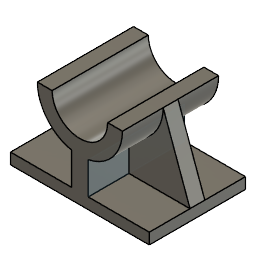
day3 (Autodesk Fusion 360 design; units mm, degrees)
part number: 2026-08-21-14-28-38-884
Autodesk Fusion 360 part; units mm, degrees
sketch "Sketch1" plane through (0, 0, 0) normal (0, 1, 0) x (1, 0, 0)
  line L0 (37.5, 26) -> (-37.5, 26)
  line L1 (-37.5, 26) -> (-37.5, -26)
  line L2 (-37.5, -26) -> (37.5, -26)
  line L3 (37.5, -26) -> (37.5, 26)
  line L4 (37.5, 26) -> (-37.5, -26) construction
  line L5 (-37.5, 26) -> (37.5, -26) construction
  dimension "d1" = 75
  dimension "d2" = 52
  constraint horizontal L0
  constraint perpendicular L0 L1
  constraint parallel L0 L2
  constraint parallel L1 L3
  constraint coincident L4 origin
  constraint coincident L5 origin
  measures "d1" distance of L1.end L2.end
  measures "d2" distance of L0.end L1.end
extrude "Extrude1" add sketch "Sketch1" along normal blind 6
sketch "Sketch2" plane through (0, 0, 26) normal (0, 0, 1) x (1, 0, 0)
  line L0 (-37.5, 0) -> (37.5, 0)
  line L1 (37.5, 0) -> (37.5, 6)
  line L2 (37.5, 6) -> (-37.5, 6)
  line L3 (-37.5, 6) -> (-37.5, 0)
  line L4 (0, 6) -> (0, 26)
  line L5 (4.5, 46) -> (-4.5, 46)
  line L6 (-4.5, 23.4445) -> (-4.5, 6)
  line L7 (-4.5, 6) -> (4.5, 6)
  line L8 (4.5, 6) -> (4.5, 23.4445)
  line L9 (0, 26) -> (-4.5, 6) construction
  line L10 (0, 26) -> (4.5, 6) construction
  line L11 (-4.5, 46) -> (-23, 46)
  line L12 (4.5, 46) -> (23, 46)
  arc A0 (-15, 46) -> (15, 46) centre (0, 46) ccw
  arc A1 (-23, 46) -> (23, 46) centre (0, 46) ccw
  dimension "d7" = 9
  dimension "d10" = 40
  dimension "d11" = 46
  dimension "d12" = 30
  constraint perpendicular L2 L4
  constraint coincident L2 L4.start
  constraint horizontal L5
  constraint perpendicular L5 L6
  constraint parallel L5 L7
  constraint parallel L6 L8
  constraint collinear L2 L7
  constraint perpendicular L6 L11
  constraint perpendicular L8 L12
  constraint coincident L12 A0.end
  constraint coincident L11 A0.start
  constraint coincident A1 L8.end
  constraint coincident A1 L6.start
  measures "d7" distance of L6.end L7.end
  measures "d10" distance of L5.end L6.end
  measures "d11" diameter of A1
  measures "d12" diameter of A0
extrude "Extrude2" add sketch "Sketch2" against normal blind 52 contours L2 L4 L6 L7 A1 | L2 L4 L7 L8 A1 | L11 L12 A0 A1
sketch "Sketch3" plane through (0, 0, 26) normal (0, 0, 1) x (1, 0, 0)
  line L0 (-37.5, 0) -> (37.5, 0)
  line L1 (37.5, 0) -> (37.5, 6)
  line L2 (37.5, 6) -> (4.5, 6)
  line L3 (4.5, 6) -> (4.5, 23.4445)
  arc A0 (4.5, 23.4445) -> (23, 46) centre (0, 46) ccw
  line L4 (23, 46) -> (15, 46)
  arc A1 (-15, 46) -> (15, 46) centre (0, 46) ccw
  line L5 (-15, 46) -> (-23, 46)
  arc A2 (-23, 46) -> (-4.5, 23.4445) centre (0, 46) ccw
  line L6 (-4.5, 23.4445) -> (-4.5, 6)
  line L7 (-4.5, 6) -> (-37.5, 6)
  line L8 (-37.5, 6) -> (-37.5, 0)
  line L9 (23, 46) -> (37.5, 6)
  constraint coincident A0.end L4.start
  constraint coincident L1.end L2.start
sketch "Sketch4" plane through (4.5, 0, 0) normal (1, 0, 0) x (0, 0, -1)
  line L0 (-26, 23.4445) -> (-26, 6)
  line L1 (-26, 6) -> (26, 6)
  line L2 (26, 6) -> (26, 23.4445)
  line L3 (26, 23.4445) -> (-26, 23.4445)
extrude "Extrude3" add sketch "Sketch3" along normal mid plane 8 from surface at -26 contours L2 L3 A0 L9
